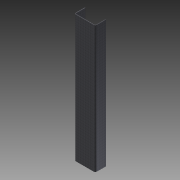
# Autodesk Inventor part: Staples
Saved by Autodesk Inventor 2011 (Build 150239000, 239)
## iProperties
Shininess: 64.0
Length Units: 11272
Angle Units: 11279
Time Units: 11290
Mass Units: 11286
Length Display Precision: 3
Angle Display Precision: 2
Compacted: True
Part Number: Staples
Document SubType Name: Modeling
Created: 2002-09-26
Designer: Autodesk, Inc.
Material: Steel, Mild
Project: Inventor Samples
Mass: 5.42321 g
Surface Area: 37.3132 cm^2
Volume: 0.689975 cm^3
Density: 7.86 g/cm^3
Density: 0.0
Volumn: 0.0
Area: 0.0
PropertySet Name: Model Information
Control State: 0
Master: False
Checked Out: False
Author: Autodesk, Inc.
Revision Number: A
Autodesk Inventor part; units mm, degrees
ref_plane "YZ Plane" through (0, 0, 0) normal (1, 0, 0) x (0, 1, 0)
ref_plane "XZ Plane" through (0, 0, 0) normal (0, 1, 0) x (-1, 0, 0)
ref_plane "XY Plane" through (0, 0, 0) normal (0, 0, 1) x (1, 0, 0)
sketch "Sketch1" plane through (0, 0, 0) normal (0, 0, 1) x (1, 0, 0)
  line L0 (0, 53.34) -> (0, -53.34) projected
  line L1 (-8.89, 0) -> (8.89, 0) projected
  line L2 (-6.35, 38.1) -> (6.35, 38.1)
  line L3 (6.35, 38.1) -> (6.35, -38.1)
  line L4 (6.35, -38.1) -> (-6.35, -38.1)
  line L5 (-6.35, -38.1) -> (-6.35, 38.1)
  dimension "d0" = 12.7
  dimension "d1" = 76.2
  constraints: 8 end point, 2 parallel, 1 horizontal, 1 perpendicular, 2 other
  measures "d0" distance of L2.start L2.end
  measures "d1" distance of L2.end L3.end
extrude "Extrusion1" add sketch "Sketch1" along normal blind 6.35
shell "Shell1" thickness 0.381 removed faces 3 at (2.1167, -38.1, 2.1167) at (2.1167, -12.7, 0) at (-2.1167, 38.1, 2.1167)
fillet "Fillet1" radius 0.508 2 edges at (-5.969, 0, 5.969) (5.969, 0, 5.969)
fillet "Fillet1" radius 1.016 2 edges at (-6.35, 0, 6.35) (6.35, 0, 6.35)
body "Solid1"
